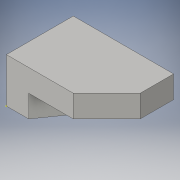
# Autodesk Inventor part: Unit 7.1 part 4
Saved by Autodesk Inventor 2016 (Build 200138000, 138)
## iProperties
Created: 2017-03-03
Part Number: Unit 7.1 part 4
Material: Generic
Document SubType Name: Modeling
Designer: 196918
Density: 1 g/cm^3
Appearance: Default
Author: 196918
Autodesk Inventor part; units mm, degrees
ref_plane "YZ Plane" through (0, 0, 0) normal (1, 0, 0) x (0, 1, 0)
ref_plane "XZ Plane" through (0, 0, 0) normal (0, 1, 0) x (-1, 0, 0)
ref_plane "XY Plane" through (0, 0, 0) normal (0, 0, 1) x (1, 0, 0)
sketch "Sketch1" plane through (0, 0, 0) normal (0, 0, 1) x (1, 0, 0)
  line L0 (0, 0) -> (57.15, 0)
  line L1 (57.15, 0) -> (57.15, 25.4)
  line L2 (57.15, 25.4) -> (0, 25.4)
  line L3 (0, 25.4) -> (0, 0)
  dimension "d0" = 57.15
  dimension "d1" = 25.4
  constraints: 8 end point, 3 perpendicular, 1 horizontal
  measures "d0" distance of L0.start L0.end
  measures "d1" distance of L0.end L1.end
extrude "Extrusion1" add sketch "Sketch1" along normal blind 38.1
sketch "Sketch2" plane through (0, 0, 38.1) normal (0, 0, 1) x (1, 0, 0)
  point P0 (0, 0)
sketch "Sketch3" plane through (0, 0, 38.1) normal (0, 0, 1) x (1, 0, 0)
  line L0 (57.355, 0) -> (57.15, 12.7)
  line L1 (57.15, 0) -> (57.15, 25.4) projected
  line L2 (57.15, 12.7) -> (12.7, 12.7)
  line L3 (12.7, 12.7) -> (12.7, 0)
  line L4 (0, 0) -> (57.15, 0) projected
  line L5 (57.15, 0) -> (12.7, 0)
  dimension "d4" = 44.45
  constraints: 8 end point, 2 perpendicular, 1 collinear, 1 midpoint, 1 point on line
  measures "d4" distance of L0.end L2.end
extrude "Extrusion2" cut sketch "Sketch3" against normal blind 38.1
draft "FaceDraft1" angle 35 pull direction (0, 0, 1) faces at (12.7, 8.4667, 25.4) fixed edges at (12.7, 6.35, 38.1)
chamfer "Chamfer1" distance 19.05 angle 45 1 edges at (57.15, 19.05, 38.1)
body "Solid1"
